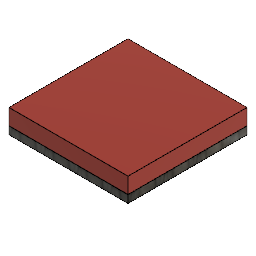
DiA_Twist-lock_base_parametric_open_source (Autodesk Fusion 360 design; units mm, degrees)
Autodesk Fusion 360 part; units mm, degrees
sketch "Twist-lock base and locker" plane through (0, 0, 0) normal (0, 0, 1) x (1, 0, 0)
  circle A0 centre (0, 0) radius 6.5
  line L0 (9, -4.5) -> (-9, -4.5)
  line L1 (-10, -3.5) -> (-10, 3.5)
  line L2 (-9, 4.5) -> (9, 4.5)
  line L3 (10, 3.5) -> (10, -3.5)
  line L4 (0, 15) -> (0, -15) construction
  line L5 (-15, 0) -> (15, 0) construction
  arc A1 (-10, -3.5) -> (-9, -4.5) centre (-9, -3.5) ccw
  arc A2 (-9, 4.5) -> (-10, 3.5) centre (-9, 3.5) ccw
  arc A3 (10, 3.5) -> (9, 4.5) centre (9, 3.5) ccw
  arc A4 (9, -4.5) -> (10, -3.5) centre (9, -3.5) ccw
  line L6 (-15, -15) -> (15, -15)
  line L7 (15, -15) -> (15, 15)
  line L8 (15, 15) -> (-15, 15)
  line L9 (-15, 15) -> (-15, -15)
  dimension "d2" = 13
  dimension "d9" = 20
  dimension "d11" = 9
  dimension "d12" = 1
  measures "d2" diameter of A0
  measures "d9" distance of L1 L3
  measures "d11" distance of L0 L2
  measures "d12" radius of A1
extrude "Extrude1" add sketch "Twist-lock base and locker" against normal blind 2 makes body 1
extrude "Extrude2" add sketch "Twist-lock base and locker" along normal blind 4 separate body contours A0 L0 L2 | A0 L0 L2 L3 A3 A4 | A0 L2 | A0 L0 | A0 L0 L1 L2 A1 A2 | L6 L7 L8 L9 makes body 2
extrude "Extrude3" add sketch "Twist-lock base and locker" against normal blind 2 contours A0 L0 L2 bodies 2
extrude "Extrude4" add sketch "Twist-lock base and locker" along normal blind -2 and the other way blind 5 contours A0 L0 L2 | A0 L0 L2 L3 A3 A4 | A0 L0 L1 L2 A1 A2 bodies 2
chamfer "Chamfer1" distance 1 angle 45 8 edges at (-10, 0, -5) (-9.7071, 4.2071, -5) (0, 4.5, -5) (9.7071, 4.2071, -5) (10, 0, -5) (9.7071, -4.2071, -5) (0, -4.5, -5) (-9.7071, -4.2071, -5) on bodies 2
sketch "Printing support" plane through (0, 4.5, 0) normal (0, 1, 0) x (-1, 0, 0)
  line L0 (-9, -4) -> (9, -4)
  line L1 (9, -4) -> (9, -2)
  line L2 (9, -2) -> (4.6904, -2)
  line L3 (4.6904, -2) -> (4.6904, 0)
  line L4 (4.6904, 0) -> (-4.6904, 0)
  line L5 (-4.6904, 0) -> (-4.6904, -2)
  line L6 (-4.6904, -2) -> (-9, -2)
  line L7 (-9, -2) -> (-9, -4)
  line L8 (4.6904, -2) -> (-4.6904, -2)
  line L9 (-4.6904, -2.4) -> (-8.6, -2.4)
  line L10 (-8.6, -2.4) -> (-8.6, -3.6)
  line L11 (-8.6, -3.6) -> (8.6, -3.6)
  line L12 (8.6, -3.6) -> (8.6, -2.4)
  line L13 (8.6, -2.4) -> (4.6904, -2.4)
  line L14 (4.6904, -2.4) -> (-4.6904, -2.4)
  dimension "d26" = 0.4
  measures "d26" distance of L6
extrude "Extrude5" add sketch "Printing support" along normal blind 10.5 separate body contours L0 L1 L2 L6 L7 L8 makes body 3
move_body "Move2" bodies 2 3 to x (0, -1, 0) y (1, 0, 0) z (0, 0, 1) at (0, 0, 0)
move_body "Move1" [rolled back]
hidden bodies 3
equation "Frame_thickness = 2 mm"
equation "Lock_thickness = 3 mm"
equation "d15 = -Frame_thickness"
equation "d19 = -Frame_thickness"
equation "d21 = -Frame_thickness"
equation "d23 = Frame_thickness + Lock_thickness"
equation "d24 = 0 °"
named bodies: "Base frame with Twist-lock hole", "Twist-lock", "Printing support"
